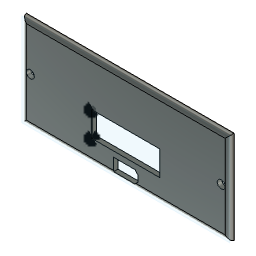
untere heckplatte (Autodesk Fusion 360 design; units mm, degrees)
Autodesk Fusion 360 part; units mm, degrees
sketch "Skizze1" plane through (0, 0, 0) normal (0, 1, 0) x (1, 0, 0)
  line L0 (0, 0) -> (90, 0)
  line L1 (90, 0) -> (90, -39)
  line L2 (90, -39) -> (0, -39)
  line L3 (0, -39) -> (0, 0)
  line L4 (0, -39) -> (2.75, -39)
  line L5 (90, -39) -> (87.25, -39)
  line L6 (2.75, -39) -> (2.75, -19.5)
  line L7 (87.25, -39) -> (87.25, -19.5)
  circle A0 centre (2.75, -19.5) radius 1.25
  circle A1 centre (87.25, -19.5) radius 1.25
  dimension "d1" = 39
  dimension "d2" = 90
  dimension "d3" = 2.75
  dimension "d4" = 2.75
  dimension "d5" = 19.5
  dimension "d6" = 19.5
  dimension "d7" = 2.5
  dimension "d8" = 2.5
  constraint horizontal L0
  constraint vertical L1
  constraint horizontal L2
  constraint vertical L3
  constraint coincident L0.start L3.end
  constraint perpendicular L3 L4
  constraint perpendicular L1 L5
  constraint perpendicular L4 L6
  constraint perpendicular L2 L7
  constraint coincident L6.end A0.centre
  constraint coincident L7.end A1.centre
  measures "d1" distance of L0.start L2.end
  measures "d2" distance of L1.end L2.end
  measures "d3" distance of L2.end L4.end
  measures "d4" distance of L1.end L5.end
  measures "d5" distance of L4.end L6.end
  measures "d6" distance of L5.end L7.end
  measures "d7" diameter of A0
  measures "d8" diameter of A1
extrude "Extrusion1" add sketch "Skizze1" along normal blind 3 makes body 1
extrude "Extrusion2" cut 1 faces at (58.7004, 3, 6.3357) along direction (0, -1, 0) blind 1 on bodies 1 bodies 1
sketch "Skizze2" plane through (0, 0, 0) normal (0, -1, 0) x (1, 0, 0)
  line L0 (2.75, 19.5) -> (45, 19.5)
  line L1 (50.5, 34.5) -> (39.5, 34.5)
  line L2 (39.5, 34.5) -> (39.5, 4.5)
  line L3 (39.5, 4.5) -> (50.5, 4.5)
  line L4 (50.5, 4.5) -> (50.5, 34.5)
  line L5 (50.5, 34.5) -> (39.5, 4.5) construction
  line L6 (39.5, 34.5) -> (50.5, 4.5) construction
  circle A0 centre (87.25, 19.5) radius 1.25
  circle A1 centre (2.75, 19.5) radius 1.25
  line L7 (90, 39) -> (0, 39)
  line L8 (0, 39) -> (0, 0)
  line L9 (0, 0) -> (90, 0)
  line L10 (90, 0) -> (90, 39)
  point P0 (45, 19.5)
  dimension "d15" = 42.25
  dimension "d16" = 11
  dimension "d17" = 30
  constraint coincident L0.start A1.centre
  constraint horizontal L1
  constraint perpendicular L1 L2
  constraint parallel L1 L3
  constraint parallel L2 L4
  constraint coincident L5 P0
  constraint coincident L6 P0
  constraint coincident P0 L0.end
  measures "d15" distance of L0.start P0
  measures "d16" distance of L2.end L3.end
  measures "d17" distance of L1.end L2.end
extrude "Extrusion3" cut sketch "Skizze2" against normal blind 8 contours L1 L2 L3 L4 bodies 1
sketch "Skizze3" plane through (0, 0, 0) normal (0, -1, 0) x (1, 0, 0)
  line L0 (39.5, 34.5) -> (50.5, 34.5)
  line L1 (50.5, 34.5) -> (50.5, 4.5)
  line L2 (50.5, 4.5) -> (39.5, 4.5)
  line L3 (39.5, 4.5) -> (39.5, 34.5)
  line L4 (90, 0) -> (79.3979, 10.6111)
  line L5 (76.5979, 16.0111) -> (82.1979, 16.0111)
  line L6 (82.1979, 16.0111) -> (82.1979, 5.2111)
  line L7 (82.1979, 5.2111) -> (76.5979, 5.2111)
  line L8 (76.5979, 5.2111) -> (76.5979, 16.0111)
  line L9 (76.5979, 16.0111) -> (82.1979, 5.2111) construction
  line L10 (82.1979, 16.0111) -> (76.5979, 5.2111) construction
  line L11 (76.5979, 5.2111) -> (77.305, 5.9182)
  line L12 (76.5979, 5.2111) -> (77.5979, 5.2111) construction
  line L13 (77.305, 5.9182) -> (76.5979, 6.6253)
  line L14 (77.305, 5.9182) -> (78.0121, 5.2111)
  line L15 (82.1979, 5.2111) -> (81.4908, 5.9182)
  line L16 (81.4908, 5.9182) -> (82.1979, 6.6253)
  line L17 (81.4908, 5.9182) -> (80.7837, 5.2111)
  circle A0 centre (87.25, 19.5) radius 1.25
  circle A1 centre (2.75, 19.5) radius 1.25
  line L18 (90, 39) -> (0, 39)
  line L19 (0, 39) -> (0, 0)
  line L20 (0, 0) -> (90, 0)
  line L21 (90, 0) -> (90, 39)
  point P0 (79.3979, 10.6111)
  dimension "d22" = 15
  dimension "d23" = 5.6
  dimension "d24" = 10.8
  dimension "d25" = 45
  dimension "d26" = 1
  dimension "d27" = 1
  constraint horizontal L5
  constraint perpendicular L5 L6
  constraint parallel L5 L7
  constraint parallel L6 L8
  constraint coincident L9 P0
  constraint coincident L10 P0
  constraint coincident P0 L4.end
  constraint horizontal L12
  constraint coincident L8 L13.end
  constraint perpendicular L11 L13
  constraint coincident L7 L14.end
  constraint perpendicular L11 L14
  constraint parallel L14 L15
  constraint coincident L6 L16.end
  constraint perpendicular L15 L16
  constraint coincident L7 L17.end
  constraint perpendicular L15 L17
  measures "d22" distance of L4.start P0
  measures "d23" distance of L6.end L7.end
  measures "d24" distance of L5.end L6.end
  measures "d25" angle of L11 L12
  measures "d26" distance of L7.end L11.end
  measures "d27" distance of L6.end L15.end
extrude "Extrusion4" cut sketch "Skizze3" against normal blind 122 contours L5 L6 L7 L8 L13 L14 L16 L17 bodies 1
sketch "Skizze4" plane through (0, 2, 0) normal (0, 1, 0) x (-1, 0, 0)
  line L0 (-78.0121, 5.2111) -> (-80.7837, 5.2111)
  line L1 (-80.7837, 5.2111) -> (-82.1979, 6.6253)
  line L2 (-82.1979, 6.6253) -> (-82.1979, 16.0111)
  line L3 (-82.1979, 16.0111) -> (-76.5979, 16.0111)
  line L4 (-76.5979, 16.0111) -> (-76.5979, 6.6253)
  line L5 (-76.5979, 6.6253) -> (-78.0121, 5.2111)
  line L6 (-50.5, 34.5) -> (-39.5, 34.5)
  line L7 (-39.5, 34.5) -> (-39.5, 4.5)
  line L8 (-39.5, 4.5) -> (-50.5, 4.5)
  line L9 (-50.5, 4.5) -> (-50.5, 34.5)
  circle A0 centre (-87.25, 19.5) radius 1.25
  circle A1 centre (-2.75, 19.5) radius 1.25
  line L10 (0, 39) -> (0, 40)
  line L11 (0, 0) -> (0, -1)
  line L12 (-90, 39) -> (-90, 40)
  line L13 (-90, 0) -> (-90, -1)
  line L14 (-90, 40) -> (0, 40)
  line L15 (-90, -1) -> (0, -1)
  line L16 (0, 39) -> (-90, 39)
  line L17 (-90, 39) -> (-90, 0)
  line L18 (-90, 0) -> (0, 0)
  line L19 (0, 0) -> (0, 39)
  dimension "d30" = 1
  dimension "d31" = 1
  dimension "d32" = 1
  dimension "d33" = 1
  measures "d30" distance of L10.start L10.end
  measures "d31" distance of L11.start L11.end
  measures "d32" distance of L12.start L12.end
  measures "d33" distance of L13.start L13.end
extrude "Extrusion5" add sketch "Skizze4" against normal blind 2 separate body contours L10 L12 L14 L16 | L11 L13 L15 L18 makes body 2 at (30, 1.3333, 39) makes body 3 at (60, 1.3333, -1)
sketch "Skizze5" plane through (0, 0, 0) normal (0, -1, 0) x (1, 0, 0)
  line L0 (0, 0) -> (90, 0)
  line L1 (90, 39) -> (0, 39)
  line L2 (39.5, 34.5) -> (50.5, 34.5)
  line L3 (50.5, 34.5) -> (50.5, 4.5)
  line L4 (50.5, 4.5) -> (39.5, 4.5)
  line L5 (39.5, 4.5) -> (39.5, 34.5)
  line L6 (80.7837, 5.2111) -> (78.0121, 5.2111)
  line L7 (78.0121, 5.2111) -> (76.5979, 6.6253)
  line L8 (76.5979, 6.6253) -> (76.5979, 16.0111)
  line L9 (76.5979, 16.0111) -> (82.1979, 16.0111)
  line L10 (82.1979, 16.0111) -> (82.1979, 6.6253)
  line L11 (82.1979, 6.6253) -> (80.7837, 5.2111)
  circle A0 centre (2.75, 19.5) radius 1.75
  circle A1 centre (87.25, 19.5) radius 1.75
  circle A2 centre (87.25, 19.5) radius 1.25
  circle A3 centre (2.75, 19.5) radius 1.25
  line L12 (0, 39) -> (0, 0)
  line L13 (90, 0) -> (90, 39)
  dimension "d38" = 3.5
  dimension "d39" = 3.5
  constraint concentric A0 A3
  constraint concentric A1 A2
  measures "d38" diameter of A0
  measures "d39" diameter of A1
extrude "Extrusion6" cut sketch "Skizze5" against normal blind 10 contours A0 | A1 | A2 | A3 bodies 1
extrude "Extrusion7" add 3 faces at (0, 1.3333, 26) (0, 1.3333, 39.3333) (0, 1.3333, -0.3333) along direction (-1, 0, 0) blind 1 on bodies 1 2 3 bodies 1 2 3
extrude "Extrusion8" add 1 faces at (90, 1.3333, 12.6667) along direction (1, 0, 0) blind 1 on bodies 1 bodies 1
sketch "Skizze6" plane through (0, 0, 0) normal (0, -1, 0) x (1, 0, 0)
  circle A0 centre (2.75, 19.5) radius 1.75
  circle A1 centre (87.25, 19.5) radius 1.75
  line L0 (80.7837, 5.2111) -> (78.0121, 5.2111)
  line L1 (78.0121, 5.2111) -> (76.5979, 6.6253)
  line L2 (76.5979, 6.6253) -> (76.5979, 16.0111)
  line L3 (76.5979, 16.0111) -> (82.1979, 16.0111)
  line L4 (82.1979, 16.0111) -> (82.1979, 6.6253)
  line L5 (82.1979, 6.6253) -> (80.7837, 5.2111)
  line L6 (39.5, 34.5) -> (50.5, 34.5)
  line L7 (50.5, 34.5) -> (50.5, 4.5)
  line L8 (50.5, 4.5) -> (39.5, 4.5)
  line L9 (39.5, 4.5) -> (39.5, 34.5)
  line L10 (-1, -1) -> (91, -1)
  line L11 (91, -1) -> (91, 40)
  line L12 (91, 40) -> (-1, 40)
  line L13 (-1, 40) -> (-1, -1)
  line L14 (39.5, 34.5) -> (39.5, 37.5)
  line L15 (39.5, 37.5) -> (50.5, 37.5)
  line L16 (50.5, 37.5) -> (50.5, 34.5)
  line L17 (39.5, 4.5) -> (39.5, 7.5)
  line L18 (39.5, 7.5) -> (50.5, 7.5)
  dimension "d46" = 3
  dimension "d47" = 3
  constraint coincident L6.start L9.end
  constraint perpendicular L6 L14
  constraint perpendicular L7 L15
  constraint coincident L6.end L7.start
  constraint perpendicular L6 L16
  constraint coincident L8.end L9.start
  constraint perpendicular L8 L17
  constraint coincident L7 L18.end
  constraint perpendicular L7 L18
  measures "d46" distance of L6.start L14.end
  measures "d47" distance of L8.end L17.end
extrude "Extrusion9" cut sketch "Skizze6" against normal blind 10 contours L6 L14 L15 L16 | L7 L8 L9 L17 L18 bodies 1
sketch "Skizze7" plane through (0, 0, 0) normal (0, -1, 0) x (1, 0, 0)
  line L0 (50.5, 37.5) -> (50.5, 4.5)
  line L1 (50.5, 4.5) -> (39.5, 4.5)
  line L2 (39.5, 4.5) -> (39.5, 37.5)
  line L3 (39.5, 37.5) -> (50.5, 37.5)
  circle A0 centre (2.75, 19.5) radius 1.75
  circle A1 centre (87.25, 19.5) radius 1.75
  line L4 (80.7837, 5.2111) -> (78.0121, 5.2111)
  line L5 (78.0121, 5.2111) -> (76.5979, 6.6253)
  line L6 (76.5979, 6.6253) -> (76.5979, 16.0111)
  line L7 (76.5979, 16.0111) -> (82.1979, 16.0111)
  line L8 (82.1979, 16.0111) -> (82.1979, 6.6253)
  line L9 (82.1979, 6.6253) -> (80.7837, 5.2111)
  line L10 (-1, -1) -> (91, -1)
  line L11 (91, -1) -> (91, 40)
  line L12 (91, 40) -> (-1, 40)
  line L13 (-1, 40) -> (-1, -1)
  line L14 (39.5, 4.5) -> (39.5, 7.5)
  line L15 (39.5, 7.5) -> (50.5, 7.5)
  dimension "d50" = 3
  constraint coincident L1.end L2.start
  constraint perpendicular L1 L14
  constraint coincident L0 L15.end
  constraint perpendicular L0 L15
  measures "d50" distance of L1.end L14.end
extrude "Extrusion10" add sketch "Skizze7" against normal blind 2 contours L0 L1 L2 L14 L15 bodies 1
sketch "Skizze8" plane through (0, 0, 0) normal (0, -1, 0) x (1, 0, 0)
  line L0 (50.5, 37.5) -> (50.5, 7.5)
  line L1 (50.5, 7.5) -> (39.5, 7.5)
  line L2 (39.5, 7.5) -> (39.5, 37.5)
  line L3 (39.5, 37.5) -> (50.5, 37.5)
  circle A0 centre (2.75, 19.5) radius 1.75
  circle A1 centre (87.25, 19.5) radius 1.75
  line L4 (80.7837, 5.2111) -> (78.0121, 5.2111)
  line L5 (78.0121, 5.2111) -> (76.5979, 6.6253)
  line L6 (76.5979, 6.6253) -> (76.5979, 16.0111)
  line L7 (76.5979, 16.0111) -> (82.1979, 16.0111)
  line L8 (82.1979, 16.0111) -> (82.1979, 6.6253)
  line L9 (82.1979, 6.6253) -> (80.7837, 5.2111)
  line L10 (-1, -1) -> (91, -1)
  line L11 (91, -1) -> (91, 40)
  line L12 (91, 40) -> (-1, 40)
  line L13 (-1, 40) -> (-1, -1)
  line L14 (39.5, 7.5) -> (39.5, 6.5)
  line L15 (39.5, 6.5) -> (39.6, 6.5)
  line L16 (39.6, 6.5) -> (39.6, 0.9)
  line L17 (39.6, 6.5) -> (50.4, 6.5)
  line L18 (39.6, 0.9) -> (50.4, 0.9)
  line L19 (50.4675, 6.5) -> (50.4675, 0.9)
  line L20 (50.4675, 0.9) -> (49.7604, 1.6071)
  line L21 (39.7383, 40) -> (39.7383, 38.5)
  line L22 (39.5, 37.5) -> (39.5, 38.5)
  line L23 (39.5, 38.5) -> (50.5, 38.5)
  line L24 (50.5, 38.5) -> (50.5, 37.5)
  dimension "d53" = 1
  dimension "d54" = 0.1
  dimension "d55" = 5.6
  dimension "d56" = 10.8
  dimension "d57" = 45
  dimension "d58" = 1
  dimension "d59" = 1.5
  dimension "d60" = 1
  dimension "d61" = 11
  constraint coincident L1.end L2.start
  constraint perpendicular L1 L14
  constraint horizontal L15
  constraint perpendicular L1 L16
  constraint perpendicular L16 L17
  constraint perpendicular L16 L18
  constraint perpendicular L18 L19
  constraint coincident L12 L21.start
  constraint perpendicular L12 L21
  constraint coincident L2.end L3.start
  constraint perpendicular L3 L22
  constraint perpendicular L21 L23
  constraint coincident L0.start L3.end
  measures "d53" distance of L1.end L14.end
  measures "d54" distance of L14.end L15.end
  measures "d55" distance of L15.end L16.end
  measures "d56" distance of L15.end L17.end
  measures "d57" angle of L19 L20
  measures "d58" distance of L19.end L20.end
  measures "d59" distance of L21.start L21.end
  measures "d60" distance of L2.end L22.end
  measures "d61" distance of L22.end L23.end
extrude "Extrusion11" cut sketch "Skizze8" against normal blind 3 contours L3 L22 L23 L24 bodies 1
sketch "Skizze9" plane through (0, 0, 0) normal (0, -1, 0) x (1, 0, 0)
  line L0 (50.5, 38.5) -> (50.5, 7.5)
  line L1 (50.5, 7.5) -> (39.5, 7.5)
  line L2 (39.5, 7.5) -> (39.5, 38.5)
  line L3 (39.5, 38.5) -> (50.5, 38.5)
  circle A0 centre (2.75, 19.5) radius 1.75
  circle A1 centre (87.25, 19.5) radius 1.75
  line L4 (80.7837, 5.2111) -> (78.0121, 5.2111)
  line L5 (78.0121, 5.2111) -> (76.5979, 6.6253)
  line L6 (76.5979, 6.6253) -> (76.5979, 16.0111)
  line L7 (76.5979, 16.0111) -> (82.1979, 16.0111)
  line L8 (82.1979, 16.0111) -> (82.1979, 6.6253)
  line L9 (82.1979, 6.6253) -> (80.7837, 5.2111)
  line L10 (-1, -1) -> (91, -1)
  line L11 (91, -1) -> (91, 40)
  line L12 (91, 40) -> (-1, 40)
  line L13 (-1, 40) -> (-1, -1)
  line L14 (44, -1) -> (44, 0.5)
  line L15 (39.5, 7.5) -> (39.6, 7.5)
  line L16 (50.5, 7.5) -> (50.4, 7.5)
  line L17 (39.6, 7.5) -> (39.6, -1)
  line L18 (39.6, 6.1) -> (50.4, 6.1)
  line L19 (39.6, 0.5) -> (50.4, 0.5)
  line L20 (50.4, 0.5) -> (50.4, 6.1)
  dimension "d64" = 1.5
  dimension "d66" = 0.1
  dimension "d67" = 0.1
  dimension "d68" = 10.8
  dimension "d69" = 10.8
  constraint coincident L10 L14.start
  constraint perpendicular L10 L14
  constraint coincident L1.end L2.start
  constraint horizontal L15
  constraint coincident L0.end L1.start
  constraint horizontal L16
  constraint coincident L10 L17.end
  constraint perpendicular L10 L17
  constraint coincident L17 L18.start
  constraint coincident L17 L19.start
  constraint perpendicular L14 L19
  constraint perpendicular L18 L20
  measures "d64" distance of L14.start L14.end
  measures "d66" distance of L1.end L15.end
  measures "d67" distance of L0.end L16.end
  measures "d68" distance of L18.start L18.end
  measures "d69" distance of L19.start L19.end
extrude "Extrusion12" cut sketch "Skizze9" against normal blind 3 contours L17 L18 L19 L20 bodies 1
sketch "Skizze10" plane through (0, 0, 0) normal (0, -1, 0) x (1, 0, 0)
  line L0 (50.4, 0.5) -> (39.6, 0.5)
  line L1 (39.6, 0.5) -> (39.6, 6.1)
  line L2 (39.6, 6.1) -> (50.4, 6.1)
  line L3 (50.4, 6.1) -> (50.4, 0.5)
  line L4 (50.5, 38.5) -> (50.5, 7.5)
  line L5 (50.5, 7.5) -> (39.5, 7.5)
  line L6 (39.5, 7.5) -> (39.5, 38.5)
  line L7 (39.5, 38.5) -> (50.5, 38.5)
  circle A0 centre (2.75, 19.5) radius 1.75
  circle A1 centre (87.25, 19.5) radius 1.75
  line L8 (80.7837, 5.2111) -> (78.0121, 5.2111)
  line L9 (78.0121, 5.2111) -> (76.5979, 6.6253)
  line L10 (76.5979, 6.6253) -> (76.5979, 16.0111)
  line L11 (76.5979, 16.0111) -> (82.1979, 16.0111)
  line L12 (82.1979, 16.0111) -> (82.1979, 6.6253)
  line L13 (82.1979, 6.6253) -> (80.7837, 5.2111)
  line L14 (-1, -1) -> (91, -1)
  line L15 (91, -1) -> (91, 40)
  line L16 (91, 40) -> (-1, 40)
  line L17 (-1, 40) -> (-1, -1)
  line L18 (50.4, 0.5) -> (49.6929, 1.2071)
  line L19 (50.4, 0.5) -> (51.4, 0.5) construction
  line L20 (49.6929, 1.2071) -> (48.9858, 0.5)
  line L21 (48.9858, 0.5) -> (50.4, 1.9142)
  line L22 (50.4, 1.9142) -> (48.9858, 0.5)
  line L23 (50.4, 6.1) -> (49.6929, 5.3929)
  line L24 (49.6929, 5.3929) -> (48.9858, 6.1)
  line L25 (49.6929, 5.3929) -> (50.4, 4.6858)
  dimension "d72" = 135
  dimension "d73" = 1
  dimension "d74" = 1
  dimension "d75" = 1
  constraint horizontal L19
  constraint coincident L0.start L3.end
  constraint coincident L0 L20.end
  constraint perpendicular L18 L20
  constraint coincident L3 L21.end
  constraint perpendicular L18 L21
  constraint coincident L2.end L3.start
  constraint parallel L22 L23
  constraint coincident L2 L24.end
  constraint coincident L3 L25.end
  constraint perpendicular L23 L25
  measures "d72" angle of L18 L19
  measures "d73" distance of L0.start L18.end
  measures "d74" distance of L2.end L23.end
  measures "d75" distance of L23.end L24.end
extrude "Extrusion13" add sketch "Skizze10" against normal blind 2 contours L3 L18 L21 L22 | L0 L18 L20 L21 L22 | L3 L23 L25 | L2 L23 L24 bodies 1
sketch "Skizze11" plane through (0, 0, 0) normal (0, -1, 0) x (1, 0, 0)
  line L0 (48.9858, 0.5) -> (39.6, 0.5)
  line L1 (39.6, 0.5) -> (39.6, 6.1)
  line L2 (39.6, 6.1) -> (48.9858, 6.1)
  line L3 (48.9858, 6.1) -> (50.4, 4.6858)
  line L4 (50.4, 4.6858) -> (50.4, 1.9142)
  line L5 (50.4, 1.9142) -> (48.9858, 0.5)
  line L6 (50.5, 38.5) -> (50.5, 7.5)
  line L7 (50.5, 7.5) -> (39.5, 7.5)
  line L8 (39.5, 7.5) -> (39.5, 38.5)
  line L9 (39.5, 38.5) -> (50.5, 38.5)
  circle A0 centre (2.75, 19.5) radius 1.75
  circle A1 centre (87.25, 19.5) radius 1.75
  line L10 (80.7837, 5.2111) -> (78.0121, 5.2111)
  line L11 (78.0121, 5.2111) -> (76.5979, 6.6253)
  line L12 (76.5979, 6.6253) -> (76.5979, 16.0111)
  line L13 (76.5979, 16.0111) -> (82.1979, 16.0111)
  line L14 (82.1979, 16.0111) -> (82.1979, 6.6253)
  line L15 (82.1979, 6.6253) -> (80.7837, 5.2111)
  line L16 (-1, -1) -> (91, -1)
  line L17 (91, -1) -> (91, 40)
  line L18 (91, 40) -> (-1, 40)
  line L19 (-1, 40) -> (-1, -1)
sketch "Skizze12" plane through (0, 0, 0) normal (0, -1, 0) x (1, 0, 0)
extrude "Extrusion14" add sketch "Skizze11" against normal blind 2 contours L10 L11 L12 L13 L14 L15 bodies 1
sketch "Skizze13" plane through (0, 0, 0) normal (0, -1, 0) x (1, 0, 0)
  line L0 (48.9858, 0.5) -> (39.6, 0.5)
  line L1 (39.6, 0.5) -> (39.6, 6.1)
  line L2 (39.6, 6.1) -> (48.9858, 6.1)
  line L3 (48.9858, 6.1) -> (50.4, 4.6858)
  line L4 (50.4, 4.6858) -> (50.4, 1.9142)
  line L5 (50.4, 1.9142) -> (48.9858, 0.5)
  line L6 (50.5, 38.5) -> (50.5, 7.5)
  line L7 (50.5, 7.5) -> (39.5, 7.5)
  line L8 (39.5, 7.5) -> (39.5, 38.5)
  line L9 (39.5, 38.5) -> (50.5, 38.5)
  circle A0 centre (2.75, 19.5) radius 1.75
  circle A1 centre (87.25, 19.5) radius 1.75
  line L10 (-1, -1) -> (91, -1)
  line L11 (91, -1) -> (91, 40)
  line L12 (91, 40) -> (-1, 40)
  line L13 (-1, 40) -> (-1, -1)
  line L14 (45, 7.5) -> (60, 7.5)
  line L15 (45, 7.5) -> (30, 7.5)
  line L16 (30, 7.5) -> (30, 18.5)
  line L17 (30, 18.5) -> (60, 18.5)
  line L18 (60, 18.5) -> (60, 7.5)
  dimension "d80" = 15
  dimension "d81" = 15
  dimension "d82" = 11
  constraint midpoint L7 L14.start
  constraint parallel L7 L14
  constraint parallel L7 L15
  constraint perpendicular L15 L16
  constraint perpendicular L6 L17
  constraint perpendicular L14 L18
  measures "d80" distance of L14.start L14.end
  measures "d81" distance of L14.start L15.end
  measures "d82" distance of L15.end L16.end
extrude "Extrusion15" cut sketch "Skizze13" against normal blind 3 contours L6 L14 L17 L18 | L8 L15 L16 L17 bodies 1
sketch "Skizze14" plane through (0, 0, 0) normal (0, -1, 0) x (1, 0, 0)
  line L0 (-1, -1) -> (91, -1)
  line L1 (91, -1) -> (91, 40)
  line L2 (91, 40) -> (-1, 40)
  line L3 (-1, 40) -> (-1, -1)
  circle A0 centre (87.25, 19.5) radius 1.75
  circle A1 centre (2.75, 19.5) radius 1.75
  line L4 (50.5, 18.5) -> (60, 18.5)
  line L5 (60, 18.5) -> (60, 7.5)
  line L6 (60, 7.5) -> (30, 7.5)
  line L7 (30, 7.5) -> (30, 18.5)
  line L8 (30, 18.5) -> (39.5, 18.5)
  line L9 (39.5, 18.5) -> (39.5, 38.5)
  line L10 (39.5, 38.5) -> (50.5, 38.5)
  line L11 (50.5, 38.5) -> (50.5, 18.5)
  line L12 (48.9858, 0.5) -> (39.6, 0.5)
  line L13 (39.6, 0.5) -> (39.6, 6.1)
  line L14 (39.6, 6.1) -> (48.9858, 6.1)
  line L15 (48.9858, 6.1) -> (50.4, 4.6858)
  line L16 (50.4, 4.6858) -> (50.4, 1.9142)
  line L17 (50.4, 1.9142) -> (48.9858, 0.5)
  line L18 (39.5, 18.5) -> (50.5, 18.5)
  constraint coincident L8.end L9.start
  constraint coincident L4.start L11.end
extrude "Extrusion16" add sketch "Skizze14" against normal blind 2 contours L9 L10 L11 L18 bodies 1
sketch "Skizze15" plane through (0, 0, 0) normal (0, -1, 0) x (1, 0, 0)
  line L0 (-1, -1) -> (91, -1)
  line L1 (91, -1) -> (91, 40)
  line L2 (91, 40) -> (-1, 40)
  line L3 (-1, 40) -> (-1, -1)
  circle A0 centre (87.25, 19.5) radius 1.75
  circle A1 centre (2.75, 19.5) radius 1.75
  line L4 (30, 18.5) -> (60, 18.5)
  line L5 (60, 18.5) -> (60, 7.5)
  line L6 (60, 7.5) -> (30, 7.5)
  line L7 (30, 7.5) -> (30, 18.5)
  line L8 (48.9858, 0.5) -> (39.6, 0.5)
  line L9 (39.6, 0.5) -> (39.6, 6.1)
  line L10 (39.6, 6.1) -> (48.9858, 6.1)
  line L11 (48.9858, 6.1) -> (50.4, 4.6858)
  line L12 (50.4, 4.6858) -> (50.4, 1.9142)
  line L13 (50.4, 1.9142) -> (48.9858, 0.5)
  line L14 (30, 18.5) -> (30, 19.5)
  line L15 (30, 19.5) -> (60, 19.5)
  line L16 (60, 19.5) -> (60, 18.5)
  dimension "d87" = 1
  constraint coincident L4.start L7.end
  constraint perpendicular L4 L14
  constraint perpendicular L14 L15
  constraint coincident L4.end L5.start
  measures "d87" distance of L4.start L14.end
extrude "Extrusion17" cut sketch "Skizze15" against normal blind 3 contours L4 L14 L15 L16 bodies 1
sketch "Skizze16" plane through (0, 0, 0) normal (0, -1, 0) x (1, 0, 0)
  line L0 (60, 19.5) -> (60, 18.5)
  line L1 (60, 18.5) -> (60, 7.5)
  line L2 (60, 7.5) -> (30, 7.5)
  line L3 (30, 7.5) -> (30, 19.5)
  line L4 (30, 19.5) -> (60, 19.5)
  line L5 (-1, -1) -> (91, -1)
  line L6 (91, -1) -> (91, 40)
  line L7 (91, 40) -> (-1, 40)
  line L8 (-1, 40) -> (-1, -1)
  circle A0 centre (87.25, 19.5) radius 1.75
  circle A1 centre (2.75, 19.5) radius 1.75
  line L9 (48.9858, 0.5) -> (39.6, 0.5)
  line L10 (39.6, 0.5) -> (39.6, 6.1)
  line L11 (39.6, 6.1) -> (48.9858, 6.1)
  line L12 (48.9858, 6.1) -> (50.4, 4.6858)
  line L13 (50.4, 4.6858) -> (50.4, 1.9142)
  line L14 (50.4, 1.9142) -> (48.9858, 0.5)
  line L15 (30, 7.5) -> (30, 8.5)
  line L16 (30, 8.5) -> (60, 8.5)
  dimension "d90" = 1
  constraint coincident L2.end L3.start
  constraint perpendicular L2 L15
  constraint coincident L1 L16.end
  constraint perpendicular L1 L16
  measures "d90" distance of L2.end L15.end
extrude "Extrusion18" add sketch "Skizze16" against normal blind 2 contours L1 L2 L3 L15 L16 bodies 1
sketch "Skizze17" plane through (0, 0, 0) normal (0, -1, 0) x (1, 0, 0)
  line L0 (60, 19.5) -> (60, 18.5)
  line L1 (60, 18.5) -> (60, 8.5)
  line L2 (60, 8.5) -> (30, 8.5)
  line L3 (30, 8.5) -> (30, 19.5)
  line L4 (30, 19.5) -> (60, 19.5)
  line L5 (-1, -1) -> (91, -1)
  line L6 (91, -1) -> (91, 40)
  line L7 (91, 40) -> (-1, 40)
  line L8 (-1, 40) -> (-1, -1)
  circle A0 centre (87.25, 19.5) radius 1.75
  circle A1 centre (2.75, 19.5) radius 1.75
  line L9 (48.9858, 0.5) -> (39.6, 0.5)
  line L10 (39.6, 0.5) -> (39.6, 6.1)
  line L11 (39.6, 6.1) -> (48.9858, 6.1)
  line L12 (48.9858, 6.1) -> (50.4, 4.6858)
  line L13 (50.4, 4.6858) -> (50.4, 1.9142)
  line L14 (50.4, 1.9142) -> (48.9858, 0.5)
  line L15 (30, 8.5) -> (30, 19.5)
  constraint coincident L2.end L3.start
  constraint coincident L3.end L4.start
fillet "Abrundung3" radius 2 4 edges at (45, 0, 40) (91, 0, 19.5) (45, 0, -1) (-1, 0, 19.5) on bodies 1
